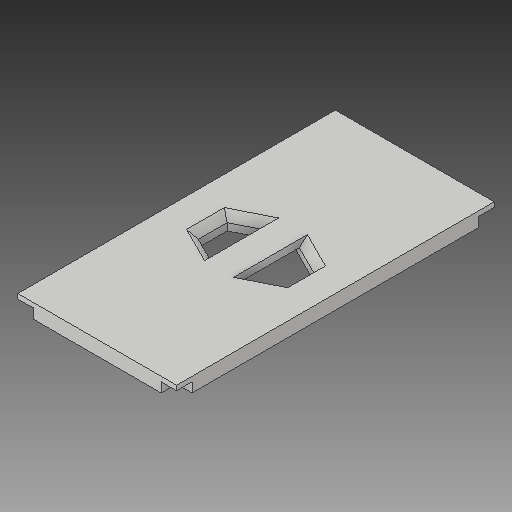
# Autodesk Inventor part: BODY_TOP_COVER
Saved by Autodesk Inventor 2017.3 (Build 213256000, 256)
## iProperties
Created: 2018-01-04
Part Number: BODY_TOP_COVER
Material: Generic
Document SubType Name: Modeling
Designer: Alex
Density: 1 g/cm^3
Appearance: Default
Author: Alex
Autodesk Inventor part; units mm, degrees
ref_plane "YZ Plane" through (0, 0, 0) normal (1, 0, 0) x (0, 1, 0)
ref_plane "XZ Plane" through (0, 0, 0) normal (0, 1, 0) x (-1, 0, 0)
ref_plane "XY Plane" through (0, 0, 0) normal (0, 0, 1) x (1, 0, 0)
sketch "Sketch1" plane through (0, 0, 0) normal (0, 1, 0) x (-1, 0, 0)
  line L0 (-27.5, 55) -> (27.5, 55)
  line L1 (27.5, 55) -> (27.5, -55)
  line L2 (27.5, -55) -> (-27.5, -55)
  line L3 (-27.5, -55) -> (-27.5, 55)
  point P0 (0, 0)
  point P1 (0, -55)
  point P2 (27.5, 0)
  dimension "d0" = 110
  dimension "d1" = 55
  constraints: 8 end point, 2 midpoint, 2 parallel, 1 horizontal, 1 horizontal alignment, 1 perpendicular, 1 vertical alignment
  measures "d0" distance of L0.end L1.end
  measures "d1" distance of L0.start L0.end
extrude "Extrusion1" add sketch "Sketch1" along normal blind 5
sketch "Sketch2" plane through (0, 0, 0) normal (0, -1, 0) x (1, 0, 0)
  line L0 (27.5, 49.65) -> (22.15, 49.65)
  line L1 (22.15, 49.65) -> (22.15, 55)
  line L2 (22.15, 55) -> (27.5, 55)
  line L3 (27.5, 55) -> (27.5, 49.65)
  line L4 (27.5, -55) -> (27.5, 55) projected
  line L5 (27.5, 55) -> (-27.5, 55) projected
  line L6 (0, -77) -> (0, 77) projected
  line L7 (-38.5, 0) -> (38.5, 0) projected
  line L8 (27.5, -49.65) -> (22.15, -49.65)
  line L9 (22.15, -49.65) -> (22.15, -55)
  line L10 (22.15, -55) -> (27.5, -55)
  line L11 (27.5, -55) -> (27.5, -49.65)
  line L12 (-27.5, 49.65) -> (-22.15, 49.65)
  line L13 (-22.15, 49.65) -> (-22.15, 55)
  line L14 (-22.15, 55) -> (-27.5, 55)
  line L15 (-27.5, 55) -> (-27.5, 49.65)
  line L16 (-22.15, -49.65) -> (-22.15, -55)
  line L17 (-27.5, -49.65) -> (-22.15, -49.65)
  line L18 (-27.5, -55) -> (-27.5, -49.65)
  line L19 (-22.15, -55) -> (-27.5, -55)
  point P0 (0, 0)
  dimension "d4" = 5.35
  constraints: 32 end point, 12 symmetric about line, 2 collinear, 2 parallel, 2 perpendicular, 1 horizontal
  measures "d4" distance of L0.start L0.end
extrude "Extrusion2" cut sketch "Sketch2" against normal blind 3.35 contours L0 L1 L2 L3 | L10 L9 L8 L4 | L13 L12 L15 L5 | L16 L19 L18 L17
sketch "Sketch3" plane through (0, 5, 0) normal (0, 1, 0) x (1, 0, 0)
  line L0 (-5, -10) -> (-15, -5)
  line L1 (-15, -5) -> (-15, 5)
  line L2 (-15, 5) -> (-5, 10)
  line L3 (-5, 10) -> (-5, -10)
  line L4 (15, -5) -> (15, 5)
  line L5 (15, 5) -> (5, 10)
  line L6 (5, 10) -> (5, -10)
  line L7 (5, -10) -> (15, -5)
  point P0 (0, 0)
  point P1 (-5, 0)
  dimension "d7" = 5
  dimension "d8" = 5
  dimension "d9" = 10
  dimension "d10" = 20
  dimension "d11" = 10
  dimension "d12" = 10
  constraints: 16 end point, 3 equal length, 3 horizontal alignment, 3 parallel, 1 midpoint, 1 vertical
  measures "d7" distance from line of point (0, 0) L3
  measures "d8" distance from line of point (0, 0) L6
  measures "d9" distance of L0.end L1.end
  measures "d10" distance of L2.end L0.start
  measures "d11" distance between parallel lines of L3 L1
  measures "d12" distance between parallel lines of L4 L6
extrude "Extrusion3" cut sketch "Sketch3" against normal through all
chamfer "Chamfer1" distance 2.5 angle 45 8 edges at (5, 0, 0) (-5, 0, 0) (-10, 5, 7.5) (-15, 5, 0) (-10, 5, -7.5) (10, 5, -7.5) (15, 5, 0) (10, 5, 7.5)
equation "\"d4\" = magnet_A"
equation "\"d5\" = magnet_B"
equation "\"magnet_A\" = 5.35"
equation "\"magnet_B\" = 3.35"
body "Solid1"
